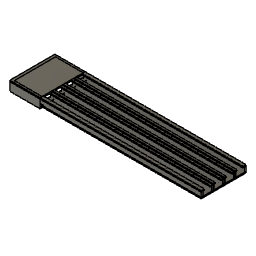
led_strip_aquarium (Autodesk Fusion 360 design; units mm, degrees)
Autodesk Fusion 360 part; units mm, degrees
note: some values were not read from the file. Set by a fixed rule: which sketch regions a step uses.
sketch "Esquisse1" plane through (0, 0, 0) normal (0, 0, 1) x (1, 0, 0)
  line L0 (0, 0) -> (250, 0)
  line L1 (250, 0) -> (250, 18.9)
  line L2 (250, 18.9) -> (0, 18.9)
  line L3 (0, 18.9) -> (0, 0)
  line L4 (0, 18.9) -> (250, 18.9)
  line L5 (250, 18.9) -> (250, 15.9)
  line L6 (250, 15.9) -> (0, 15.9)
  line L7 (0, 15.9) -> (0, 18.9)
  line L8 (0, 0) -> (250, 0)
  line L9 (250, 0) -> (250, 3)
  line L10 (250, 3) -> (0, 3)
  line L11 (0, 3) -> (0, 0)
  line L12 (0, 3) -> (250, 3)
  line L13 (250, 3) -> (250, 4.9)
  line L14 (250, 4.9) -> (0, 4.9)
  line L15 (0, 4.9) -> (0, 3)
  line L16 (0, 15.9) -> (250, 15.9)
  line L17 (250, 15.9) -> (250, 14)
  line L18 (250, 14) -> (0, 14)
  line L19 (0, 14) -> (0, 15.9)
  line L20 (0, 9.45) -> (250, 9.45)
  line L21 (0, 9.45) -> (16.4793, 9.45)
  line L22 (250, 9.45) -> (90, 9.45)
  line L23 (0, 9.45) -> (45.5008, 9.45)
  line L24 (125, 4.9) -> (125, 14)
  circle A0 centre (16.4793, 9.45) radius 2.25
  circle A1 centre (31.0011, 9.45) radius 2.25
  circle A2 centre (45.5008, 9.45) radius 2.25
  circle A3 centre (60.001, 9.45) radius 2.25
  circle A4 centre (74.5003, 9.45) radius 2.25
  circle A5 centre (89.0664, 9.45) radius 2.25
  circle A6 centre (103.5817, 9.45) radius 2.25
  circle A7 centre (118.0077, 9.45) radius 2.25
  circle A8 centre (131.9923, 9.45) radius 2.25
  circle A9 centre (146.4183, 9.45) radius 2.25
  circle A10 centre (160.9336, 9.45) radius 2.25
  circle A11 centre (175.4997, 9.45) radius 2.25
  circle A12 centre (189.999, 9.45) radius 2.25
  circle A13 centre (204.4992, 9.45) radius 2.25
  circle A14 centre (218.9989, 9.45) radius 2.25
  circle A15 centre (233.5207, 9.45) radius 2.25
  dimension "d1" = 250
  dimension "d2" = 18.9
  dimension "d3" = 3
  dimension "d4" = 3
  dimension "d5" = 1.9
  dimension "d6" = 1.9
  dimension "d63" = 4.5
  dimension "d64" = 4.5
  dimension "d65" = 4.5
  dimension "d66" = 4.5
  dimension "d67" = 4.5
  dimension "d68" = 4.5
  dimension "d69" = 4.5
  dimension "d70" = 4.5
  constraint horizontal L0
  constraint vertical L1
  constraint horizontal L2
  constraint vertical L3
  constraint coincident L0.start L3.end
  constraint horizontal L4
  constraint vertical L5
  constraint horizontal L6
  constraint vertical L7
  constraint horizontal L8
  constraint vertical L9
  constraint horizontal L10
  constraint vertical L11
  constraint horizontal L12
  constraint vertical L13
  constraint horizontal L14
  constraint vertical L15
  constraint horizontal L16
  constraint vertical L17
  constraint horizontal L18
  constraint vertical L19
  constraint midpoint L3 L20.start
  constraint perpendicular L1 L20
  constraint coincident L1 L9.end
  constraint midpoint L1 L20.end
  constraint coincident L1 L5.end
  constraint perpendicular L3 L21
  constraint coincident L20 L22.end
  constraint perpendicular L3 L23
  constraint midpoint L14 L24.start
  constraint midpoint L18 L24.end
  constraint coincident L21.end A0.centre
  constraint coincident L23 A1.centre
  constraint coincident L23.end A2.centre
  constraint coincident L20 A3.centre
  constraint coincident L20 A4.centre
  constraint coincident L20 A5.centre
  constraint coincident L20 A6.centre
  constraint coincident L22 A7.centre
  constraint symmetric L24 A0 A15
  constraint symmetric L24 A1 A14
  constraint symmetric L24 A2 A13
  constraint symmetric L24 A3 A12
  constraint symmetric L24 A4 A11
  constraint symmetric L24 A5 A10
  constraint symmetric L24 A6 A9
  constraint symmetric L24 A7 A8
  measures "d1" distance of L0.start L0.end
  measures "d2" distance of L0.start L2.end
  measures "d3" distance of L2.end L6.end
  measures "d4" distance of L0.start L10.end
  measures "d5" distance of L10.end L14.end
  measures "d6" distance of L6.end L18.end
  measures "d63" diameter of A0
  measures "d64" diameter of A1
  measures "d65" diameter of A2
  measures "d66" diameter of A3
  measures "d67" diameter of A4
  measures "d68" diameter of A5
  measures "d69" diameter of A6
  measures "d70" diameter of A7
extrude "Extrusion3" add sketch "Esquisse1" along normal blind 2 makes body 1
extrude "Extrusion2" add sketch "Esquisse1" along normal blind 9.5 separate body contours L0 L1 L3 L8 L9 L10 L11 L12 | L1 L2 L3 L4 L5 L6 L7 L16 makes body 2 at (166.6667, 18.9, 3.1667) makes body 3 at (166.6667, 3, 3.1667)
extrude "Extrusion1" add sketch "Esquisse1" along normal blind 2 separate body contours L0 L1 L3 L8 L9 L10 L11 L12 | L1 L3 L10 L12 L13 L14 L15 | L1 L3 L6 L16 L17 L18 L19 | L1 L2 L3 L4 L5 L6 L7 L16 makes body 4 at (166.6667, 15.6333, 0) makes body 5 at (83.3333, 1.6333, 0)
move_body "Déplacer1" bodies 5 4 to x (1, 0, 0) y (0, 1, 0) z (0, 0, 1) at (0, 0, 9)
sketch "Esquisse2" plane through (0, 0, 9.5) normal (0, 0, 1) x (-1, 0, 0) in component "Component"
  line L0 (0, 29.1) -> (0, 34)
  line L1 (0, 34) -> (-250, 34)
  line L2 (-250, 34) -> (-250, 29.1)
  line L3 (-250, 29.1) -> (0, 29.1)
  line L4 (0, 34) -> (47, 34)
  line L5 (47, 34) -> (47, -35.9)
  line L6 (47, -35.9) -> (0, -35.9)
  line L7 (0, -35.9) -> (0, 34)
  line L8 (0, 31) -> (43, 31)
  line L9 (43, 31) -> (43, -32.9)
  line L10 (43, -32.9) -> (0, -32.9)
  line L11 (0, -32.9) -> (0, 31)
  line L12 (0, 31) -> (4, 31)
  line L13 (4, 31) -> (4, -32.9)
  line L14 (4, -32.9) -> (0, -32.9)
  line L15 (0, -32.9) -> (0, 31)
  line L16 (0, 34) -> (-5, 34)
  line L17 (-5, 34) -> (-5, -35.9)
  line L18 (-5, -35.9) -> (0, -35.9)
  line L19 (0, -35.9) -> (0, 34)
  line L20 (35.0121, -32.9) -> (22.2621, -32.9)
  line L21 (43, -32.9) -> (22, -32.9)
  line L22 (43, -1.4) -> (43, -32.9)
  line L23 (22, 2.5) -> (22, -0.5)
  line L24 (43, -4.4) -> (43, -1.4)
  line L25 (22, 2.5) -> (25, 2.5)
  line L26 (25, -29) -> (22, -29)
  dimension "d36" = 47
  dimension "d37" = 43
  dimension "d38" = 63.9
  dimension "d43" = 4
  dimension "d77" = 31.5
  dimension "d78" = 3
  dimension "d81" = 69.9
  dimension "d82" = 69.9
  constraint horizontal L4
  constraint vertical L5
  constraint horizontal L6
  constraint vertical L7
  constraint coincident L0.end L1.start
  constraint horizontal L8
  constraint vertical L9
  constraint horizontal L10
  constraint vertical L11
  constraint coincident L7 L8.start
  constraint horizontal L12
  constraint vertical L13
  constraint horizontal L14
  constraint vertical L15
  constraint horizontal L16
  constraint vertical L17
  constraint horizontal L18
  constraint vertical L19
  constraint coincident L10 L20.start
  constraint horizontal L21
  constraint vertical L22
  constraint vertical L23
  constraint vertical L24
  constraint horizontal L25
  constraint horizontal L26
  measures "d36" distance of L0.end L4.end
  measures "d37" distance of L8.start L8.end
  measures "d38" distance of L8.start L10.end
  measures "d43" distance of L8.start L12.end
  measures "d77" distance of L9.end L22.start
  measures "d78" distance of L22.start L24.start
  measures "d81" distance of L4.end L5.end
  measures "d82" distance of L16.end L17.end
extrude "Extrusion4" add sketch "Esquisse2" against normal blind 15 separate body contours L0 L4 L5 L6 L7 L8 L9 L10 L12 L14 L19 L20 L21 L22 L24 makes body 6 in component "Component"
extrude "Extrusion3'" add sketch "Esquisse2" against normal blind 2 separate body contours L0 L7 L8 L10 L11 L12 L13 L14 L15 L19 | L0 L4 L5 L6 L7 L8 L9 L10 L12 L14 L19 L20 L21 L22 L24 | L8 L9 L10 L13 L20 L21 L22 L24 makes body 7 in component "Component"
extrude "Extrusion5" add sketch "Esquisse2" against normal blind 7.5 from surface at -7.5 separate body contours L0 L1 L3 L7 L11 L15 L16 L17 L19 | L3 L7 L11 L15 L17 L18 L19 | L0 L7 L8 L10 L11 L12 L13 L14 L15 L19 makes body 8 in component "Component"
chamfer "Chanfrein1" distance 3 angle 45 1 edges at (-4, 0.95, 2) on bodies 8 in component "Component"
hole "Perçage2" at (-33.4418, 35.9, 1.0038) direction (0, -1, 0) diameter 11 depth 11 tip angle 90 bodies 6 in component "Component"
chamfer "Chanfrein2" distance 5 angle 45 1 edges at (5, 0.95, -5.5) on bodies 8 in component "Component"
extrude "Extrusion5'" cut sketch "Esquisse1" along normal blind 5 contours L20 L21 L23 A0 | L20 L21 L23 A0 | L20 L22 A7 | L20 L22 A7 | L20 L23 A1 | L20 L23 A1 | L20 L22 A6 | L20 L22 A6 | L20 L23 A2 | L20 L23 A2 | L20 L22 A5 | L20 L22 A5 | L20 A3 | L20 A3 | L20 A4 | L20 A4 bodies 1
extrude "Extrusion6" cut sketch "Esquisse1" along normal blind 5 contours L20 L22 A15 | L20 L22 A15 | L20 L22 A8 | L20 L22 A8 | L20 L22 A14 | L20 L22 A14 | L20 L22 A9 | L20 L22 A9 | L20 L22 A13 | L20 L22 A13 | L20 L22 A10 | L20 L22 A10 | L20 L22 A12 | L20 L22 A12 | L20 L22 A11 | L20 L22 A11 bodies 1
move_body "Déplacer1'" bodies 8 6 7 to x (1, 0, 0) y (0, 1, 0) z (0, 0, 1) at (0, 0, 1.5) in component "Component"
copy_body "CopyPasteBodies9" bodies 4 3 2 1 5 makes body 9 makes body 10 makes body 11 makes body 12 makes body 13
move_body "Déplacer10" bodies 9 10 11 12 13 to x (1, 0, 0) y (0, 1, 0) z (0, 0, 1) at (0, 17, 0)
copy_body "CopyPasteBodies10" bodies 5 4 3 2 1 makes body 14 makes body 15 makes body 16 makes body 17 makes body 18
move_body "Déplacer11" bodies 14 15 16 17 18 to x (1, 0, 0) y (0, 1, 0) z (0, 0, 1) at (0, -34, 0)
copy_body "CopyPasteBodies11" bodies 1 2 3 4 5 makes body 19 makes body 20 makes body 21 makes body 22 makes body 23
move_body "Déplacer12" bodies 19 20 21 22 23 to x (1, 0, 0) y (0, 1, 0) z (0, 0, 1) at (0, -17, 0)
component "Component" placed x (1, 0, 0) y (0, 1, 0) z (0, 0, 1) at (0, 0, 0)
